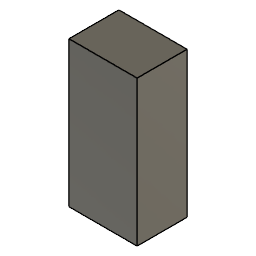
flipdot-spacers (Autodesk Fusion 360 design; units mm, degrees)
Autodesk Fusion 360 part; units mm, degrees
sketch "Sketch1" plane through (0, 0, 0) normal (0, 0, 1) x (1, 0, 0)
  line L0 (7.5, -5.5) -> (-7.5, -5.5)
  line L1 (-7.5, -5.5) -> (-7.5, 5.5)
  line L2 (-7.5, 5.5) -> (7.5, 5.5)
  line L3 (7.5, 5.5) -> (7.5, -5.5)
  line L4 (7.5, -5.5) -> (-7.5, 5.5) construction
  line L5 (-7.5, -5.5) -> (7.5, 5.5) construction
  dimension "d1" = 15
  dimension "d2" = 11
  constraint horizontal L0
  constraint perpendicular L0 L1
  constraint parallel L0 L2
  constraint parallel L1 L3
  constraint coincident L4 origin
  constraint coincident L5 origin
  measures "d1" distance of L1.end L2.end
  measures "d2" distance of L0.end L1.end
extrude "Extrude1" add sketch "Sketch1" along normal blind 32
